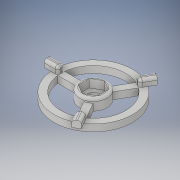
# Autodesk Inventor part: Screw
Saved by Autodesk Inventor 2019 (Build 230136000, 136)
## iProperties
Created: 2018-06-22
Part Number: Screw
Material: Ogólny
Document SubType Name: Modeling
Designer: Kamil
Density: 1 g/cm^3
Appearance: Domyślna
Author: Kamil
Autodesk Inventor part; units mm, degrees
ref_plane "YZ Plane" through (0, 0, 0) normal (1, 0, 0) x (0, 1, 0)
ref_plane "XZ Plane" through (0, 0, 0) normal (0, 1, 0) x (-1, 0, 0)
ref_plane "XY Plane" through (0, 0, 0) normal (0, 0, 1) x (1, 0, 0)
sketch "Szkic1" plane through (0, 0, 0) normal (0, 1, 0) x (-1, 0, 0)
  circle A0 centre (0, 0) radius 28.5
  line L0 (7, -4.041452) -> (0, -8.082904)
  line L1 (0, -8.082904) -> (-1.341362, -7.308468)
  line L2 (-7, -4.041452) -> (-7, 4.041452)
  line L3 (-7, 4.041452) -> (-5.909433, 4.671091)
  line L4 (0, 8.082904) -> (7, 4.041452)
  line L5 (7, 4.041452) -> (7, 2.5)
  line L6 (-1.341362, 7.308468) -> (15.026073, 7.308468) construction
  line L7 (-5.909433, 4.671091) -> (10.425295, 4.671091) construction
  line L8 (-5.909433, -4.671091) -> (10.425295, -4.671091) construction
  line L9 (-1.217256, -7.38012) -> (15.134448, -7.38012) construction
  line L10 (-5.67987, 4.803629) -> (10.684937, 4.803629) construction
  line L11 (-1.341362, -7.308468) -> (-1.382731, -7.38012)
  line L12 (-1.341362, -7.308468) -> (15.026073, -7.308468) construction
  line L13 (-5.67987, -4.803629) -> (10.684937, -4.803629) construction
  arc A1 (23.366643, 2.5) -> (-9.52508, 21.483083) centre (0, 0) ccw
  arc A2 (23.366643, -2.5) -> (23.366643, 2.5) centre (0, 0) ccw
  line L14 (7, -2.5) -> (7, -4.041452)
  line L15 (7, 2.5) -> (7, -2.5)
  line L16 (-1.341362, -7.308468) -> (-5.67987, -4.803629)
  line L17 (-5.67987, -4.803629) -> (-5.909433, -4.671091)
  arc A3 (-9.52508, -21.483083) -> (23.366643, -2.5) centre (0, 0) ccw
  arc A4 (-13.862274, -18.975968) -> (-9.52508, -21.483083) centre (0, 0) ccw
  line L18 (-1.341362, 7.308468) -> (0, 8.082904)
  line L19 (-2.683548, 9.633201) -> (-9.52508, 21.483083)
  line L20 (-7.018884, 7.122869) -> (-13.862274, 18.975968)
  line L21 (-5.909433, 4.671091) -> (-1.341362, 7.308468)
  line L22 (9.682458, 2.5) -> (23.366643, 2.5)
  arc A5 (8.841997, -4.671091) -> (9.682458, -2.5) centre (0, 0) ccw
  line L23 (-2.683548, -9.633201) -> (-9.52508, -21.483083)
  arc A6 (-13.862274, 18.975968) -> (-13.862274, -18.975968) centre (0, 0) ccw
  line L24 (-7.018884, -7.122869) -> (-7.167408, -7.38012)
  line L25 (-7, -7.090161) -> (-7.018884, -7.122869)
  arc A7 (-2.683548, -9.633201) -> (8.841997, -4.671091) centre (0, 0) ccw
  line L26 (-5.909433, -4.671091) -> (-7, -4.041452)
  arc A8 (-7.018884, 7.122869) -> (-7.018884, -7.122869) centre (0, 0) ccw
  line L27 (-7.167408, -7.38012) -> (-13.862274, -18.975968)
  arc A9 (-2.684658, -9.632892) -> (-2.683548, -9.633201) centre (0, 0) ccw
  line L28 (9.682458, -2.5) -> (23.366643, -2.5)
  arc A10 (9.682458, 2.5) -> (-2.683548, 9.633201) centre (0, 0) ccw
  line L29 (9.669873, -2.5) -> (9.682458, -2.5)
  point P0 (7, 0)
  point P1 (-13.862274, 18.975968)
  point P2 (-13.862274, 18.975968)
  dimension "d0" = 57
  constraints: 60 end point, 32 point on circle, 22 coincident, 12 point on line, 11 centre point, 9 horizontal, 2 parallel, 13 other
  measures "d0" diameter of A0
extrude "Wyciągnięcie proste1" add sketch "Szkic1" along normal blind 5 contours A0 | A2 L28 A9 L22 | A9 A5 A7 A8 | A4 L27 L24 A9 L23
sketch "Szkic2" plane through (0, 5, 0) normal (0, 1, 0) x (1, 0, 0)
  line L0 (9.52523, -21.483301) -> (13.862343, -18.976056)
  line L1 (13.862343, -18.976056) -> (18.867151, -27.633532)
  line L2 (18.867151, -27.633532) -> (14.530039, -30.140777)
  line L3 (14.530039, -30.140777) -> (9.52523, -21.483301)
  line L4 (13.862343, 18.976054) -> (9.52523, 21.48353)
  line L5 (9.52523, 21.48353) -> (14.530384, 30.140806)
  line L6 (14.530384, 30.140806) -> (18.867496, 27.63333)
  line L7 (18.867496, 27.63333) -> (13.862343, 18.976054)
  line L8 (-23.367877, -2.497003) -> (-23.367877, 2.499407)
  line L9 (-23.367877, 2.499407) -> (-33.367877, 2.499407)
  line L10 (-33.367877, 2.499407) -> (-33.367877, -2.497003)
  line L11 (-33.367877, -2.497003) -> (-23.367877, -2.497003)
  point P0 (0, 0)
  dimension "d14" = 10
  dimension "d15" = 10
  dimension "d16" = 10
  constraints: 24 end point, 6 parallel, 3 perpendicular, 1 vertical
  measures "d14" distance of L0.end L1.end
  measures "d15" distance of L4.end L5.end
  measures "d16" distance of L9.end L8.end
extrude "Wyciągnięcie proste2" add sketch "Szkic2" along normal blind 5
sketch "Szkic3" plane through (0, 0, 0) normal (0, -1, 0) x (1, 0, 0)
  line L0 (7, -4.041452) -> (0, -8.082904)
  line L1 (0, -8.082904) -> (-7, -4.041452)
  line L2 (-7, -4.041452) -> (-7, 4.041452)
  line L3 (-7, 4.041452) -> (0, 8.082904)
  line L4 (0, 8.082904) -> (7, 4.041452)
  line L5 (7, 4.041452) -> (7, -4.041452)
  circle A0 centre (0, 0) radius 4
  point P0 (7, 0)
  dimension "d19" = 8
  constraints: 12 end point, 2 coincident, 1 centre point, 1 midpoint, 13 other
  measures "d19" diameter of A0
extrude "Wyciągnięcie proste3" add sketch "Szkic3" against normal blind 2
sketch "Szkic4" plane through (0, 5, 0) normal (0, 1, 0) x (1, 0, 0)
  circle A0 centre (0, 0) radius 10
  line L0 (-7, 4.041452) -> (0, 8.082904)
  line L1 (0, 8.082904) -> (7, 4.041452)
  line L2 (7, 4.041452) -> (7, -4.041452)
  line L3 (7, -4.041452) -> (0, -8.082904)
  line L4 (0, -8.082904) -> (-7, -4.041452)
  line L5 (-7, -4.041452) -> (-7, 4.041452)
  point P0 (-7, 0)
  dimension "d22" = 20
  constraints: 12 end point, 2 coincident, 1 centre point, 1 midpoint, 13 other
  measures "d22" diameter of A0
extrude "Wyciągnięcie proste4" add sketch "Szkic4" along normal blind 3
fillet "Zaokrąglenie1" radius 2 1 edges at (16.3647, 10, 23.3048)
fillet "Zaokrąglenie2" radius 2 3 edges at (10.828, 10, 20.7302) (13.3552, 9.4142, 19.2692) (13.8623, 6.5, 18.9761)
fillet "Zaokrąglenie3" radius 2 3 edges at (12.5281, 10, 26.6778) (9.8184, 9.4142, 21.9904) (9.5252, 6.5, 21.4833)
fillet "Zaokrąglenie4" radius 2 1 edges at (-28.3679, 10, 2.497)
fillet "Zaokrąglenie5" radius 2 3 edges at (-23.3679, 10, -1.0012) (-23.3679, 9.4142, 1.9112) (-23.3679, 6.5, 2.497)
fillet "Zaokrąglenie6" radius 2 3 edges at (-29.3679, 10, -2.4994) (-23.9537, 9.4142, -2.4994) (-23.3679, 6.5, -2.4994)
fillet "Zaokrąglenie7" radius 2 1 edges at (16.3649, 10, -23.3047)
fillet "Zaokrąglenie8" radius 2 3 edges at (10.8281, 10, -20.7303) (13.3552, 9.4142, -19.2692) (13.8623, 6.5, -18.9761)
fillet "Zaokrąglenie9" radius 2 3 edges at (12.5283, 10, -26.6779) (9.8184, 9.4142, -21.9907) (9.5252, 6.5, -21.4835)
fillet "Zaokrąglenie10" radius 2 1 edges at (-10, 8, 0)
